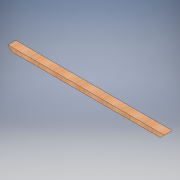
# Autodesk Inventor part: Right Panel Front 45 Diagonal Piece
Saved by Autodesk Inventor 2016 (Build 200138000, 138)
## iProperties
Created: 2015-07-05
Part Number: Right Panel Front 45 Diagonal Piece
Material: Wood (Birch)
Document SubType Name: Modeling
Designer: steele
Density: 0.55 g/cm^3
Appearance: Birch - Natural Polished
Author: steele
Autodesk Inventor part; units mm, degrees
ref_plane "YZ Plane" through (0, 0, 0) normal (1, 0, 0) x (0, 1, 0)
ref_plane "XZ Plane" through (0, 0, 0) normal (0, 1, 0) x (-1, 0, 0)
ref_plane "XY Plane" through (0, 0, 0) normal (0, 0, 1) x (1, 0, 0)
sketch "Sketch2" plane through (0, 0, 0) normal (0, 0, 1) x (1, 0, 0)
  line L0 (-830.9741, -22.6629) -> (830.9741, -22.6629)
  line L1 (876.3, 22.6629) -> (-876.3, 22.6629)
  line L2 (-876.3, -22.6629) -> (876.3, 22.6629) construction
  line L3 (876.3, -22.6629) -> (-876.3, 22.6629) construction
  line L4 (-876.3, 22.6629) -> (-830.9741, -22.6629)
  line L5 (-876.3, 22.6629) -> (-812.1996, 22.6629) construction
  line L6 (876.3, 22.6629) -> (830.9741, -22.6629)
  line L7 (876.3, 22.6629) -> (940.4004, 22.6629) construction
  point P0 (0, 0)
  dimension "d10" = 45
  dimension "d11" = 135
  dimension "d14" = 1752.6
  constraints: 16 end point, 3 horizontal, 2 equal length, 2 midpoint, 1 parallel
  measures "d10" angle of L4 L5
  measures "d11" angle of L6 L7
  measures "d14" distance of L1.start L1.end
extrude "Extrusion2" add sketch "Sketch2" along normal mid plane 88.9
body "Solid2"
